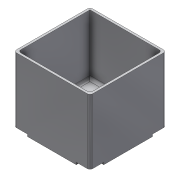
# Autodesk Inventor part: сосуд
Saved by Autodesk Inventor 2021 (Build 250183000, 183)
## iProperties
Created: 2023-02-14
Part Number: сосуд
Material: Типовые
Document SubType Name: Modeling
Designer: Tasya
Density: 1 g/cm^3
Appearance: Гладкий - белый
Author: Tasya
Autodesk Inventor part; units mm, degrees
ref_plane "YZ Plane" through (0, 0, 0) normal (1, 0, 0) x (0, 1, 0)
ref_plane "XZ Plane" through (0, 0, 0) normal (0, 1, 0) x (-1, 0, 0)
ref_plane "XY Plane" through (0, 0, 0) normal (0, 0, 1) x (1, 0, 0)
sketch "Эскиз1" plane through (0, 0, 0) normal (0, 1, 0) x (-1, 0, 0)
  line L0 (-70.5, 70.5) -> (70.5, 70.5)
  line L1 (70.5, 70.5) -> (70.5, -70.5)
  line L2 (70.5, -70.5) -> (-70.5, -70.5)
  line L3 (-70.5, -70.5) -> (-70.5, 70.5)
  line L4 (-70.5, 70.5) -> (70.5, -70.5) construction
  line L5 (70.5, 70.5) -> (-70.5, -70.5) construction
  point P0 (0, 0)
  dimension "d0" = 141
  constraints: 12 end point, 2 midpoint, 2 parallel, 2 perpendicular, 1 horizontal
  measures "d0" distance of L0.end L1.end
extrude "Выдавливание1" add sketch "Эскиз1" along normal blind 120
sketch "Эскиз2" plane through (0, 120, 0) normal (0, 1, 0) x (1, 0, 0)
  line L0 (66.5, -66.5) -> (-66.5, -66.5)
  line L1 (-66.5, -66.5) -> (-66.5, 66.5)
  line L2 (-66.5, 66.5) -> (66.5, 66.5)
  line L3 (66.5, 66.5) -> (66.5, -66.5)
  line L4 (66.5, -66.5) -> (-66.5, 66.5) construction
  line L5 (-66.5, -66.5) -> (66.5, 66.5) construction
  line L6 (-70.5, 70.5) -> (-70.5, -70.5) projected
  point P0 (0, 0)
  dimension "d3" = 4
  constraints: 12 end point, 2 midpoint, 2 parallel, 2 perpendicular, 1 horizontal
  measures "d3" distance between parallel lines of L6 L1
extrude "Выдавливание2" cut sketch "Эскиз2" against normal blind 110
fillet "Сопряжение1" radius 5 11 edges at (70.5, 60, 70.5) (66.5, 65, 66.5) (70.5, 60, -70.5) (66.5, 65, -66.5) (-66.5, 65, 66.5) (-66.5, 10, 0) (0, 10, 66.5) (66.5, 10, 0) (0, 10, -66.5) (-70.5, 60, -70.5) (-70.5, 60, 70.5)
sketch "Эскиз3" plane through (0, 0, 0) normal (0, -1, 0) x (1, 0, 0)
  arc A0 (-65.5, 70.5) -> (-70.5, 65.5) centre (-65.5, 65.5) ccw projected
  line L0 (-70.5, -65.5) -> (-70.5, 65.5) projected
  arc A1 (-70.5, -65.5) -> (-65.5, -70.5) centre (-65.5, -65.5) ccw projected
  line L1 (65.5, -70.5) -> (-65.5, -70.5) projected
  arc A2 (65.5, -70.5) -> (70.5, -65.5) centre (65.5, -65.5) ccw projected
  line L2 (70.5, 65.5) -> (70.5, -65.5) projected
  arc A3 (70.5, 65.5) -> (65.5, 70.5) centre (65.5, 65.5) ccw projected
  line L3 (-65.5, 70.5) -> (65.5, 70.5) projected
  line L4 (45, -70.5) -> (-45, -70.5)
  line L5 (-45, -70.5) -> (-45, -66.5)
  line L6 (-45, -66.5) -> (45, -66.5)
  line L7 (45, -66.5) -> (45, -70.5)
  line L8 (70.5, 65.5) -> (70.5, -65.5) projected
  line L9 (70.5, -45) -> (70.5, 45)
  line L10 (70.5, 45) -> (66.5, 45)
  line L11 (66.5, 45) -> (66.5, -45)
  line L12 (66.5, -45) -> (70.5, -45)
  line L13 (-70.5, -45) -> (-70.5, 45)
  line L14 (-70.5, 45) -> (-66.5, 45)
  line L15 (-66.5, 45) -> (-66.5, -45)
  line L16 (-66.5, -45) -> (-70.5, -45)
  line L17 (-65.5, 70.5) -> (65.5, 70.5) projected
  line L18 (45, 70.5) -> (-45, 70.5)
  line L19 (-45, 70.5) -> (-45, 66.5)
  line L20 (-45, 66.5) -> (45, 66.5)
  line L21 (45, 66.5) -> (45, 70.5)
  line L22 (0, 0) -> (0, -15.64) construction
  line L23 (0, 0) -> (-17.2484, 0) construction
  point P0 (45, 70.5)
  point P1 (-45, 70.5)
  point P2 (70.5, 45)
  dimension "d7" = 4
  dimension "d8" = 90
  constraints: 36 end point, 9 point on line, 8 parallel, 6 equal length, 4 perpendicular, 1 collinear, 1 horizontal, 1 vertical, 2 other
  measures "d7" distance between parallel lines of L2 L11
  measures "d8" distance of L10.end L11.end
extrude "Выдавливание3" add sketch "Эскиз3" along normal blind 4 contours L3 L21 L20 L19 | L14 L15 L16 L0 | L2 L12 L11 L10 | L5 L6 L7 L1
